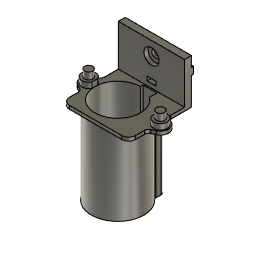
pump_holder (Autodesk Fusion 360 design; units mm, degrees)
Autodesk Fusion 360 part; units mm, degrees
sketch "Grundriss" plane through (0, 0, 0) normal (0, 0, 1) x (1, 0, 0)
  line L0 (0, 0) -> (42, 0) construction
  line L1 (42, 0) -> (42, 36) construction
  line L2 (42, 36) -> (0, 36) construction
  line L3 (0, 36) -> (0, 0) construction
  line L4 (-0.5, -0.5) -> (42.5, -0.5)
  line L5 (42.5, -0.5) -> (42.5, 36.5)
  line L6 (42.5, 36.5) -> (-0.5, 36.5) construction
  line L7 (-0.5, 36.5) -> (-0.5, -0.5)
  circle A0 centre (16, 18) radius 16 construction
  line L8 (42, 18) -> (0, 18) construction
  line L9 (-3, -3) -> (45, -3)
  line L10 (45, -3) -> (45, 39)
  line L11 (45, 39) -> (-3, 39) construction
  line L12 (-3, 39) -> (-3, -3)
  circle A1 centre (16, 18) radius 16.5
  line L13 (21, -0.5) -> (21, 36) construction
  line L14 (-7.483, 23.4621) -> (-3, 25.5)
  line L15 (-7.483, 12.5379) -> (-3, 10.5)
  arc A2 (-7.483, 23.4621) -> (-7.483, 12.5379) centre (-5, 18) ccw
  line L16 (49.483, 23.4621) -> (45, 25.5)
  arc A3 (49.483, 12.5379) -> (49.483, 23.4621) centre (47, 18) ccw
  line L17 (49.483, 12.5379) -> (45, 10.5)
  line L18 (-3, 39) -> (-3, 42.5)
  line L19 (-3, 42.5) -> (45, 42.5)
  line L20 (45, 42.5) -> (45, 39)
  line L21 (42.5, 36.5) -> (42.5, 38)
  line L22 (42.5, 38) -> (-0.5, 38)
  line L23 (-0.5, 38) -> (-0.5, 36.5)
  line L24 (16, 36.5) -> (26, 36.5)
  line L25 (26, 36.5) -> (26, 31.1244)
  line L26 (26, 31.1244) -> (16, 31.1244)
  line L27 (16, 31.1244) -> (16, 36.5)
  line L28 (16, 36.5) -> (26, 31.1244) construction
  line L29 (26, 36.5) -> (16, 31.1244) construction
  point P0 (21, 33.8122)
  dimension "d1" = 42
  dimension "d2" = 36
  dimension "d3" = 0.5
  dimension "d4" = 16
  dimension "d5" = 3
  dimension "d6" = 0.5
  dimension "d10" = 12
  dimension "d11" = 15
  dimension "d12" = 13.5
  dimension "d13" = 11.0895
  dimension "d18" = 52
  dimension "d19" = 6
  dimension "d39" = 1.5
  dimension "d46" = 10
  dimension "d47" = 1.5
  constraint horizontal L0
  constraint vertical L1
  constraint horizontal L2
  constraint vertical L3
  constraint coincident L0.start L3.end
  constraint midpoint L1 L8.start
  constraint midpoint L3 L8.end
  constraint coincident A0.centre L8
  constraint midpoint L4 L13.start
  constraint midpoint L2 L13.end
  constraint coincident L12 L14.end
  constraint coincident L12 L15.end
  constraint tangent L14 A2
  constraint tangent L15 A2
  constraint symmetric L13 L14.start L16.start
  constraint symmetric L13 L14.end L16.end
  constraint symmetric L13 L15.start A3.start
  constraint symmetric L13 L15.end L17.end
  constraint symmetric L13 A2 A3
  constraint horizontal A0.centre A2.centre
  constraint perpendicular L11 L18
  constraint perpendicular L18 L19
  constraint collinear L10 L20
  constraint perpendicular L6 L21
  constraint perpendicular L21 L22
  constraint collinear L7 L23
  constraint perpendicular L24 L25
  constraint parallel L24 L26
  constraint parallel L25 L27
  constraint horizontal L24
  constraint coincident L28 P0
  constraint coincident L29 P0
  constraint coincident L13 P0
  constraint tangent L7 A1
  constraint coincident A1 L25.end
  measures "d1" distance of L0.start L0.end
  measures "d2" distance of L0.start L2.end
  measures "d4" radius of A0
  measures "d10" diameter of A2
  measures "d11" distance of L14.end L15.end
  measures "d12" distance of L9 L15.end
  measures "d18" distance of A2.centre A3.centre
  measures "d19" distance of L6 L19
  measures "d39" distance of L6 L22
  measures "d46" distance of L24.start L24.end
  measures "d47" distance of L22 L24
extrude "Extrude1" add sketch "Grundriss" along normal blind 2.5 contours L4 L5 L7 L21 L22 L23 | L9 L10 L12 L18 L19 L20 | L12 L14 L15 A2 | L10 L16 A3 L17
sketch "Abhebung" plane through (0, 0, 2.5) normal (0, 0, 1) x (-1, 0, 0)
  line L0 (-49.483, -23.4621) -> (-45, -25.5)
  line L1 (-45, -25.5) -> (-45, -42.5)
  line L2 (-45, -42.5) -> (3, -42.5)
  line L3 (3, -42.5) -> (3, -25.5)
  line L4 (3, -25.5) -> (7.483, -23.4621)
  arc A0 (7.483, -23.4621) -> (7.483, -12.5379) centre (5, -18) ccw
  line L5 (7.483, -12.5379) -> (3, -10.5)
  line L6 (3, -10.5) -> (3, 3)
  line L7 (3, 3) -> (-45, 3)
  line L8 (-45, 3) -> (-45, -10.5)
  line L9 (-45, -10.5) -> (-49.483, -12.5379)
  arc A1 (-49.483, -12.5379) -> (-49.483, -23.4621) centre (-47, -18) ccw
  line L10 (3, -37.5) -> (-45, -37.5)
  circle A2 centre (5, -18) radius 5
  circle A3 centre (-47, -18) radius 5
  line L11 (0.5, -37.5) -> (0.5, 3)
  line L12 (-42.5, -37.5) -> (-42.5, 3)
  line L13 (-16, -34.5) -> (-16, -36.5)
  line L14 (-16, -36.5) -> (-26, -36.5)
  line L15 (-26, -36.5) -> (-26, -31.1244)
  arc A4 (-16, -34.5) -> (-26, -31.1244) centre (-16, -18) ccw
  dimension "d21" = 5
  dimension "d22" = 10
  dimension "d23" = 2.5
  dimension "d24" = 2.5
  constraint coincident L3 L10.start
  constraint coincident L1 L10.end
  constraint perpendicular L1 L10
  constraint concentric A0 A2
  constraint concentric A1 A3
  constraint equal A2 A3
  constraint coincident L10 L11.start
  constraint coincident L7 L11.end
  constraint perpendicular L7 L11
  constraint coincident L10 L12.start
  constraint coincident L7 L12.end
  constraint perpendicular L7 L12
  measures "d21" distance of L2 L10
  measures "d22" diameter of A2
  measures "d23" distance of L6 L11
  measures "d24" distance of L8 L12
extrude "Extrude3" add sketch "Abhebung" along normal blind 4 contours A3 L12 | A2 L11 picked at (-45.6481, -17.7518)
extrude "Extrude4" add sketch "Abhebung" along normal blind 30 contours L1 L2 L3 L10
sketch "Sketch4" plane through (0, 0, 6.5) normal (0, 0, 1) x (-1, 0, 0)
  arc A0 (-42.5, -15.8206) -> (-42.5, -20.1794) centre (-47, -18) ccw
  line L0 (-42.5, -20.1794) -> (-42.5, -15.8206)
  circle A1 centre (-47, -18) radius 3
  circle A2 centre (5, -18) radius 3
  arc A3 (0.5, -20.1794) -> (0.5, -15.8206) centre (5, -18) ccw
  dimension "d29" = 6
  constraint concentric A0 A1
  constraint concentric A2 A3
  constraint equal A1 A2
  measures "d29" diameter of A1
extrude "Extrude5" add sketch "Sketch4" along normal blind 5 contours A1 | A2
sketch "Montage" plane through (0, 37.5, 0) normal (0, -1, 0) x (1, 0, 0)
  line L0 (-3, 2.5) -> (45, 2.5)
  line L1 (45, 2.5) -> (45, 32.5)
  line L2 (45, 32.5) -> (-3, 32.5)
  line L3 (-3, 32.5) -> (-3, 2.5)
  line L4 (21, -0.8204) -> (21, 32.5) construction
  circle A0 centre (21, 22.5) radius 5.5
  circle A1 centre (21, 22.5) radius 2.75
  line L5 (24.25, 8.5) -> (17.75, 8.5)
  line L6 (17.75, 8.5) -> (17.75, 5.5)
  line L7 (17.75, 5.5) -> (24.25, 5.5)
  line L8 (24.25, 5.5) -> (24.25, 8.5)
  line L9 (24.25, 8.5) -> (17.75, 5.5) construction
  line L10 (17.75, 8.5) -> (24.25, 5.5) construction
  point P0 (21, 7)
  dimension "d32" = 11
  dimension "d34" = 5.5
  dimension "d40" = 6.5
  dimension "d41" = 3
  dimension "d42" = 3
  dimension "d64" = 10
  constraint midpoint L2 L4.end
  constraint coincident L4 A0.centre
  constraint concentric A0 A1
  constraint perpendicular L5 L6
  constraint parallel L5 L7
  constraint parallel L6 L8
  constraint horizontal L5
  constraint coincident L9 P0
  constraint coincident L10 P0
  constraint coincident L4 P0
  constraint perpendicular L2 L4
  measures "d32" diameter of A0
  measures "d34" diameter of A1
  measures "d40" distance of L6.end L7.end
  measures "d41" distance of L5.end L6.end
  measures "d42" distance of L0 L7
  measures "d64" distance of L2 A0.centre
extrude "Extrude6" cut sketch "Montage" against normal up to surface (5 mm away) contours A1
extrude "Extrude7" cut sketch "Montage" against normal up to surface (3 mm away) contours A0
extrude "Extrude8" cut sketch "Montage" against normal up to surface (5 mm away) contours L5 L6 L7 L8
sketch "Boden" plane through (0, 0, 0) normal (0, 0, -1) x (1, 0, 0)
  line L0 (-3, -25.5) -> (-3, -42.5)
  line L1 (-3, -42.5) -> (45, -42.5)
  line L2 (45, -42.5) -> (45, -25.5)
  line L3 (45, -25.5) -> (49.483, -23.4621)
  arc A0 (49.483, -23.4621) -> (49.483, -12.5379) centre (47, -18) ccw
  line L4 (49.483, -12.5379) -> (45, -10.5)
  line L5 (45, -10.5) -> (45, 3)
  line L6 (45, 3) -> (-3, 3)
  line L7 (-3, 3) -> (-3, -10.5)
  line L8 (-3, -10.5) -> (-7.483, -12.5379)
  arc A1 (-7.483, -12.5379) -> (-7.483, -23.4621) centre (-5, -18) ccw
  line L9 (-7.483, -23.4621) -> (-3, -25.5)
  line L10 (13.5, -39) -> (13.5, -36.8348)
  arc A2 (28.5, -32.3091) -> (13.5, -36.8348) centre (16, -18) ccw
  line L11 (28.5, -32.3091) -> (28.5, -39)
  line L12 (28.5, -39) -> (13.5, -39)
  line L13 (21, -42.5) -> (21, 3) construction
  line L14 (45, -37.5) -> (-3, -37.5)
  line L15 (16, -36.5) -> (16, -34.5)
  arc A3 (26, -31.1244) -> (16, -34.5) centre (16, -18) ccw
  line L16 (26, -31.1244) -> (26, -36.5)
  line L17 (26, -36.5) -> (16, -36.5)
  dimension "d66" = 2.5
  dimension "d67" = 2.5
  dimension "d68" = 2.5
  dimension "d69" = 2.5
  constraint midpoint L1 L13.start
  constraint midpoint L6 L13.end
  constraint perpendicular L11 L12
  constraint perpendicular L10 L12
  constraint concentric A2 A3
  measures "d66" distance of L10 L15
  measures "d67" distance of L11 L16
  measures "d68" distance of L12 L17
  measures "d69" distance of A2 A3
extrude "Extrude9" add sketch "Boden" along normal blind 58 contours L10 L11 L12 L14 | L10 A2 L11 L14
extrude "Extrude10" add sketch "Boden" along normal blind 2.5 from surface at 58 contours L10 L11 L12 L14 | L10 A2 L11 L14 | L15 A3 L16 L17
fillet "Fillet1" radius 5 2 edges at (-3, -3, 1.25) (45, -3, 1.25)
fillet "Fillet2" radius 3 4 edges at (45, 10.5, 1.25) (45, 25.5, 1.25) (-3, 10.5, 1.25) (-3, 25.5, 1.25)
fillet "Fillet3" radius 2 4 edges at (28.5, 32.3091, -30.25) (13.5, 36.8348, -30.25) (13.5, 39, -30.25) (28.5, 39, -30.25)
sketch "Sketch8" plane through (0, 42.5, 0) normal (0, 1, 0) x (-1, 0, 0)
  line L0 (-17.75, 5.5) -> (-24.25, 5.5)
  line L1 (-24.25, 5.5) -> (-24.25, 8.5)
  line L2 (-24.25, 8.5) -> (-17.75, 8.5)
  line L3 (-17.75, 8.5) -> (-17.75, 5.5)
  circle A0 centre (-21, 22.5) radius 2.75
  line L4 (-45, 0) -> (3, 0)
  line L5 (3, 0) -> (3, 32.5)
  line L6 (3, 32.5) -> (-45, 32.5)
  line L7 (-45, 32.5) -> (-45, 0)
  line L8 (-42.5, 25) -> (-45, 25)
  line L9 (-45, 25) -> (-45, 20)
  line L10 (-45, 20) -> (-42.5, 20)
  line L11 (-42.5, 20) -> (-42.5, 25)
  line L12 (-42.5, 25) -> (-45, 20) construction
  line L13 (-45, 25) -> (-42.5, 20) construction
  line L14 (0.5, 25) -> (3, 25)
  line L15 (3, 25) -> (3, 20)
  line L16 (3, 20) -> (0.5, 20)
  line L17 (0.5, 20) -> (0.5, 25)
  line L18 (0.5, 25) -> (3, 20) construction
  line L19 (3, 25) -> (0.5, 20) construction
  point P0 (-43.75, 22.5)
  point P1 (1.75, 22.5)
  dimension "d58" = 2.5
  dimension "d59" = 5
  dimension "d60" = 5
  dimension "d61" = 2.5
  constraint perpendicular L8 L9
  constraint parallel L8 L10
  constraint parallel L9 L11
  constraint horizontal L8
  constraint coincident L12 P0
  constraint coincident L13 P0
  constraint perpendicular L14 L15
  constraint parallel L14 L16
  constraint parallel L15 L17
  constraint horizontal L14
  constraint coincident L18 P1
  constraint coincident L19 P1
  constraint horizontal A0.centre P0
  constraint horizontal A0.centre P1
  constraint collinear L7 L9
  constraint collinear L5 L15
  measures "d58" distance of L9.end L10.end
  measures "d59" distance of L8.end L9.end
  measures "d60" distance of L14.end L15.end
  measures "d61" distance of L15.end L16.end
extrude "Extrude11" add sketch "Sketch8" along normal blind 1.5 contours L7 L8 L9 L10 L11 | L5 L14 L15 L16 L17
equation "d4 = ( 32 / 2 ) * 1 mm"
equation "d5 = 2.5 mm + d3"
equation "d6 = d3"
equation "d24 = d23"
equation "d61 = d58"
equation "d67 = d66"
equation "d68 = d66"
equation "d69 = d66"
